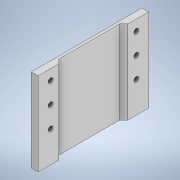
# Autodesk Inventor part: wheelguard
Saved by Autodesk Inventor 2020.1 (Build 241239000, 239)
## iProperties
Created: 2019-12-06
Part Number: wheelguard
Material: Generic
Document SubType Name: Modeling
Designer: tbloo
Density: 1 g/cm^3
Appearance: Default
Author: tbloo
Autodesk Inventor part; units mm, degrees
ref_plane "YZ Plane" through (0, 0, 0) normal (1, 0, 0) x (0, 1, 0)
ref_plane "XZ Plane" through (0, 0, 0) normal (0, 1, 0) x (-1, 0, 0)
ref_plane "XY Plane" through (0, 0, 0) normal (0, 0, 1) x (1, 0, 0)
sketch "Sketch1" plane through (0, 0, 0) normal (1, 0, 0) x (0, 1, 0)
  line L0 (0, 0) -> (64, 0)
  line L1 (64, 0) -> (64, 85)
  line L2 (64, 85) -> (0, 85)
  line L3 (0, 85) -> (0, 0)
  dimension "d0" = 64
  dimension "d1" = 85
  constraints: 8 end point, 2 parallel, 1 horizontal, 1 perpendicular
  measures "d0" distance of L2.end L1.end
  measures "d1" distance of L1.end L0.end
extrude "Extrusion1" add sketch "Sketch1" along normal blind 2
sketch "Sketch2" plane through (2, 0, 0) normal (1, 0, 0) x (0, 0, -1)
  circle A0 centre (-75.4, 56) radius 1.85 projected
  circle A1 centre (-75.4, 40) radius 1.85 projected
  circle A2 centre (-9.6, 56) radius 1.85 projected
  circle A3 centre (-9.6, 40) radius 1.85 projected
  circle A4 centre (-9.6, 24) radius 1.85 projected
  circle A5 centre (-75.4, 24) radius 1.85 projected
  line L0 (-69, 0) -> (-69, 64)
  line L1 (-69, 0) -> (-5, 0) construction
  line L2 (-16, 0) -> (-16, 64)
  line L3 (-16, 0) -> (48, 0) construction
  line L4 (-85, 64) -> (-85, 0) projected
  line L5 (-69, 64) -> (-85, 64)
  line L6 (-85, 64) -> (-85, 0)
  line L7 (-85, 0) -> (-69, 0)
  line L8 (-69, 0) -> (-69, 64)
  line L9 (0, 0) -> (0, 64) projected
  line L10 (-16, 64) -> (0, 64)
  line L11 (0, 64) -> (0, 0)
  line L12 (0, 0) -> (-16, 0)
  line L13 (-16, 0) -> (-16, 64)
  dimension "d4" = 90
  dimension "d5" = 90
  constraints: 24 end point, 4 horizontal, 4 parallel, 4 perpendicular
  measures "d4" angle of L1 L0
  measures "d5" angle of L3 L2
extrude "Extrusion2" add sketch "Sketch2" along normal blind 3.2
chamfer "Chamfer1" distance 3.175 angle 45 2 edges at (2, 32, 16) (2, 32, 69)
sketch "Sketch3" plane through (5.2, 0, 0) normal (1, 0, 0) x (0, 0, -1)
  circle A0 centre (-75.4, 56) radius 1.85 projected
  circle A1 centre (-75.4, 40) radius 1.85 projected
  circle A2 centre (-75.4, 24) radius 1.85 projected
  circle A3 centre (-9.6, 24) radius 1.85 projected
  circle A4 centre (-9.6, 40) radius 1.85 projected
  circle A5 centre (-9.6, 56) radius 1.85 projected
  point P0 (0, 0)
extrude "Extrusion3" cut sketch "Sketch3" against normal through all
body "Solid1"
